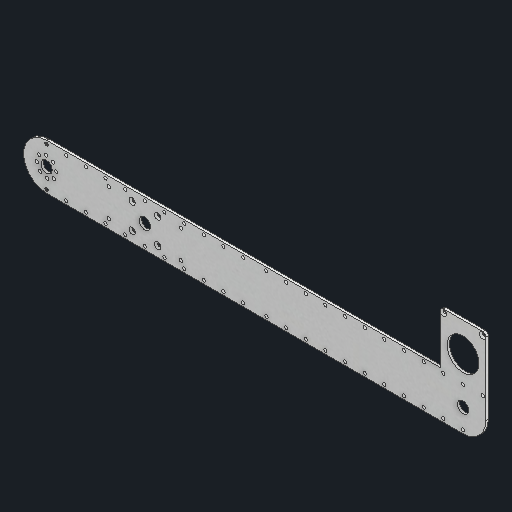
# Autodesk Inventor part: FirstStageArmBar1
Saved by Autodesk Inventor 2025 (Build 290162000, 162)
## iProperties
Created: 2023-11-22
Part Number: FirstStageArmBar1
Material: Aluminum 6061
Document SubType Name: Modeling
Designer: avsar
Density: 2.7 g/cm^3
Appearance: Paint
Mass: 273.267 g
Surface Area: 709.347 cm^2
Volume: 101.21 cm^3
Author: avsar
Autodesk Inventor part; units mm, degrees
ref_plane "YZ Plane" through (0, 0, 0) normal (1, 0, 0) x (0, 1, 0)
ref_plane "XZ Plane" through (0, 0, 0) normal (0, 1, 0) x (-1, 0, 0)
ref_plane "XY Plane" through (0, 0, 0) normal (0, 0, 1) x (1, 0, 0)
sketch "Sketch1" plane through (0, 0, 0) normal (0, 0, 1) x (1, 0, 0)
  line L0 (-254.2423, -28) -> (254.2423, -28)
  line L1 (282.2423, 0) -> (282.2423, 28)
  line L2 (282.2423, 28) -> (-254.2423, 28) construction
  line L3 (-282.2423, 0) -> (-282.2423, 0)
  line L4 (-282.2423, -28) -> (282.2423, 28) construction
  line L5 (282.2423, -28) -> (-282.2423, 28) construction
  arc A0 (-254.2423, 28) -> (-282.2423, 0) centre (-254.2423, 0) ccw
  arc A1 (-282.2423, 0) -> (-254.2423, -28) centre (-254.2423, 0) ccw
  circle A2 centre (-134.2423, 0) radius 7
  circle A3 centre (-149.7986, 15.5563) radius 2.1
  line L6 (-134.2423, 0) -> (-149.7986, 15.5563) construction
  line L7 (-134.2423, 0) -> (-254.2423, 0) construction
  circle A4 centre (-149.7986, -15.5563) radius 2.1
  circle A5 centre (-118.6859, -15.5563) radius 2.1
  circle A6 centre (-118.6859, 15.5563) radius 2.1
  arc A7 (254.2423, -28) -> (282.2423, 0) centre (254.2423, 0) ccw
  circle A8 centre (254.2423, 0) radius 7
  line L8 (282.2423, 28) -> (282.2423, 92)
  line L9 (282.2423, 92) -> (226.2423, 92)
  line L10 (226.2423, 92) -> (226.2423, 28)
  line L11 (226.2423, 28) -> (-254.2423, 28)
  circle A9 centre (254.2423, 56) radius 19.5
  circle A10 centre (-254.2423, 0) radius 7
  circle A11 centre (-263.1865, 8) radius 2
  circle A12 centre (-266.2237, -0.6677) radius 2
  circle A13 centre (-262.2423, -8.9443) radius 2
  circle A14 centre (-253.5746, -11.9814) radius 2
  circle A15 centre (-245.298, -8) radius 2
  circle A16 centre (-242.2609, 0.6677) radius 2
  circle A17 centre (-246.2423, 8.9443) radius 2
  circle A18 centre (-254.91, 11.9814) radius 2
  line L12 (-134.2423, 0) -> (254.2423, 56) construction
  point P0 (0, 0)
  point P1 (-282.2423, 0)
  dimension "d1" = 56
  dimension "d3" = 28
  dimension "d4" = 14
  dimension "d5" = 120
  dimension "d6" = 4.2
  dimension "d7" = 45
  dimension "d8" = 22
  dimension "d11" = 360
  dimension "d13" = 28
  dimension "d16" = 14
  dimension "d17" = 64
  dimension "d18" = 56
  dimension "d19" = 39
  dimension "d20" = 56
  dimension "d21" = 14
  dimension "d22" = 4
  dimension "d24" = 8
  dimension "d27" = 360
  dimension "d50" = 12
  dimension "d65" = 392.5
  constraints: 26 end point, 19 centre point, 9 point on line, 6 point on circle, 6 tangent, 3 perpendicular, 2 coincident, 2 midpoint, 2 parallel, 1 collinear, 1 concentric, 1 horizontal, 1 horizontal alignment, 1 vertical, 1 vertical alignment, 26 other
  measures "d1" distance of L4.end L5.start
  measures "d3" radius of A0
  measures "d4" diameter of A2
  measures "d5" distance of L6.start L7.end
  measures "d6" diameter of A3
  measures "d7" angle of L7 L6
  measures "d8" distance of L6.start L6.end
  measures "d13" radius of A7
  measures "d16" diameter of A8
  measures "d17" distance of L1.end L8.end
  measures "d18" distance of L8.end L9.end
  measures "d19" diameter of A9
  measures "d20" distance of L12.end A7.centre
  measures "d21" diameter of A10
  measures "d22" diameter of A11
  measures "d24" vertical distance of L7.end A11.centre
  measures "d50" distance of A11.centre L7.end
  measures "d65" distance of L6.start L12.end
extrude "Extrusion1" add sketch "Sketch1" along normal blind 3
sketch "Sketch2" plane through (0, 0, 3) normal (0, 0, 1) x (1, 0, 0)
  line L0 (226.2423, 28) -> (-254.2423, 28) construction
  circle A0 centre (-254.2423, 24) radius 2
  circle A1 centre (-230.2423, 24) radius 2
  circle A2 centre (-206.2423, 24) radius 2
  circle A3 centre (-182.2423, 24) radius 2
  circle A4 centre (-158.2423, 24) radius 2
  circle A5 centre (-134.2423, 24) radius 2
  circle A6 centre (-110.2423, 24) radius 2
  circle A7 centre (-86.2423, 24) radius 2
  circle A8 centre (-62.2423, 24) radius 2
  circle A9 centre (-38.2423, 24) radius 2
  circle A10 centre (-14.2423, 24) radius 2
  line L1 (0, 28) -> (0, -28) construction
  line L2 (-254.2423, -28) -> (254.2423, -28) construction
  circle A11 centre (254.2423, 24) radius 2
  circle A12 centre (230.2423, 24) radius 2
  circle A13 centre (206.2423, 24) radius 2
  circle A14 centre (182.2423, 24) radius 2
  circle A15 centre (158.2423, 24) radius 2
  circle A16 centre (134.2423, 24) radius 2
  circle A17 centre (110.2423, 24) radius 2
  circle A18 centre (86.2423, 24) radius 2
  circle A19 centre (62.2423, 24) radius 2
  circle A20 centre (38.2423, 24) radius 2
  circle A21 centre (14.2423, 24) radius 2
  arc A22 (-254.2423, 28) -> (-254.2423, -28) centre (-254.2423, 0) ccw construction
  arc A23 (254.2423, -28) -> (282.2423, 0) centre (254.2423, 0) ccw construction
  line L3 (-282.2423, 0) -> (282.2423, 0) construction
  line L4 (226.2423, -28) -> (-254.2423, -28) construction
  circle A24 centre (-254.2423, -24) radius 2
  circle A25 centre (-230.2423, -24) radius 2
  circle A26 centre (-206.2423, -24) radius 2
  circle A27 centre (-182.2423, -24) radius 2
  circle A28 centre (-158.2423, -24) radius 2
  circle A29 centre (-134.2423, -24) radius 2
  circle A30 centre (-110.2423, -24) radius 2
  circle A31 centre (-86.2423, -24) radius 2
  circle A32 centre (-62.2423, -24) radius 2
  circle A33 centre (-38.2423, -24) radius 2
  circle A34 centre (-14.2423, -24) radius 2
  circle A35 centre (62.2423, -24) radius 2
  circle A36 centre (38.2423, -24) radius 2
  circle A37 centre (14.2423, -24) radius 2
  circle A38 centre (86.2423, -24) radius 2
  circle A39 centre (110.2423, -24) radius 2
  circle A40 centre (134.2423, -24) radius 2
  circle A41 centre (158.2423, -24) radius 2
  circle A42 centre (182.2423, -24) radius 2
  circle A43 centre (206.2423, -24) radius 2
  circle A44 centre (230.2423, -24) radius 2
  circle A45 centre (254.2423, -24) radius 2
  circle A46 centre (230.2423, 88) radius 2.1
  line L5 (226.2423, 92) -> (226.2423, 28) construction
  line L6 (282.2423, 92) -> (226.2423, 92) construction
  circle A47 centre (278.2423, 88) radius 2.1
  line L7 (282.2423, 0) -> (282.2423, 92) construction
  circle A48 centre (278.2423, 24) radius 2.1
  point P0 (0, 0)
  point P1 (254.2423, 28)
  dimension "d29" = 4
  dimension "d30" = 4
  dimension "d33" = 24
  dimension "d38" = 4.2
  dimension "d39" = 4
  dimension "d40" = 4
  dimension "d41" = 4.2
  dimension "d42" = 4
  dimension "d43" = 4
  dimension "d56" = 4.2
  constraints: 47 centre point, 35 symmetric about line, 6 end point, 2 horizontal, 2 point on line, 2 vertical alignment, 1 horizontal alignment, 1 midpoint, 1 point on circle, 1 vertical, 53 other
  measures "d29" diameter of A0
  measures "d30" distance of L0.end A0.centre
  measures "d33" distance of A0.centre A1.centre
  measures "d38" diameter of A46
  measures "d39" distance from line of L5 A46.centre
  measures "d40" distance from line of L6 A46.centre
  measures "d41" diameter of A47
  measures "d42" distance from line of L6 A47.centre
  measures "d43" distance from line of L7 A47.centre
  measures "d56" diameter of A48
extrude "Extrusion2" cut sketch "Sketch2" against normal through all
sketch "Sketch3" plane through (0, 0, 3) normal (0, 0, 1) x (1, 0, 0)
  circle A0 centre (-134.2423, 0) radius 7 construction
  circle A1 centre (-90.2423, 17) radius 2.1
  line L0 (-134.2423, 0) -> (-127.2423, 0) construction
  circle A2 centre (-134.2423, 0) radius 7 construction
  line L1 (-134.2423, 0) -> (-134.2423, 7) construction
  circle A3 centre (-90.2423, -17) radius 2.1
  circle A4 centre (-178.2423, 17) radius 2.1
  circle A5 centre (-178.2423, -17) radius 2.1
  point P0 (0, 0)
  dimension "d51" = 4.2
  dimension "d52" = 44
  dimension "d53" = 17
  constraints: 4 centre point, 4 end point, 3 symmetric about line, 2 point on circle, 1 horizontal, 1 perpendicular, 3 other
  measures "d51" diameter of A1
  measures "d52" horizontal distance of A1.centre L0.start
  measures "d53" vertical distance of A1.centre L0.start
extrude "Extrusion3" cut sketch "Sketch3" against normal through all
fillet "Fillet1" radius 4 2 edges at (226.2423, 92, 1.5) (282.2423, 92, 1.5)
sketch "Sketch4" plane through (0, 0, 3) normal (0, 0, 1) x (1, 0, 0)
  circle A0 centre (-149.7986, 15.5563) radius 2.1 projected
  circle A1 centre (-118.6859, 15.5563) radius 2.1 projected
  circle A2 centre (-118.6859, -15.5563) radius 2.1 projected
  circle A3 centre (-149.7986, -15.5563) radius 2.1 projected
  point P0 (0, 0)
hole "Hole1" at (-149.7986, 15.5563, 3) at (-149.7986, -15.5563, 3) at (-118.6859, -15.5563, 3) at (-118.6859, 15.5563, 3) direction (0, 0, -1) diameter 4.2 end through all countersink diameter 8 countersink angle 90
sketch "Sketch5" plane through (0, 0, 0) normal (0, 0, -1) x (-1, 0, 0)
  circle A0 centre (178.2423, -17) radius 2.1 projected
  circle A1 centre (90.2423, -17) radius 2.1 projected
  circle A2 centre (90.2423, 17) radius 2.1 projected
  circle A3 centre (178.2423, 17) radius 2.1 projected
  circle A4 centre (158.2423, 24) radius 2 projected
  circle A5 centre (62.2423, 24) radius 2 projected
  circle A6 centre (62.2423, -24) radius 2 projected
  circle A7 centre (110.2423, -24) radius 2 projected
  circle A8 centre (206.2423, 24) radius 2 projected
  circle A9 centre (230.2423, -24) radius 2 projected
  circle A10 centre (-38.2423, -24) radius 2 projected
  circle A11 centre (-62.2423, -24) radius 2 projected
  circle A12 centre (-110.2423, 24) radius 2 projected
  circle A13 centre (-206.2423, 24) radius 2 projected
  circle A14 centre (-254.2423, -24) radius 2 projected
  circle A15 centre (-86.2423, -24) radius 2 projected
  circle A16 centre (-254.2423, 24) radius 2 projected
  circle A17 centre (-278.2423, 88) radius 2.1 projected
  circle A18 centre (-134.2423, 24) radius 2 projected
  circle A19 centre (-158.2423, -24) radius 2 projected
  circle A20 centre (-134.2423, -24) radius 2 projected
  circle A21 centre (-206.2423, -24) radius 2 projected
  circle A22 centre (182.2423, -24) radius 2 projected
  circle A23 centre (134.2423, -24) radius 2 projected
  circle A24 centre (38.2423, -24) radius 2 projected
  circle A25 centre (38.2423, 24) radius 2 projected
  circle A26 centre (134.2423, 24) radius 2 projected
  circle A27 centre (182.2423, 24) radius 2 projected
  circle A28 centre (86.2423, 24) radius 2 projected
  circle A29 centre (230.2423, 24) radius 2 projected
  circle A30 centre (86.2423, -24) radius 2 projected
  circle A31 centre (158.2423, -24) radius 2 projected
  circle A32 centre (206.2423, -24) radius 2 projected
  circle A33 centre (-182.2423, -24) radius 2 projected
  circle A34 centre (-62.2423, 24) radius 2 projected
  circle A35 centre (-86.2423, 24) radius 2 projected
  circle A36 centre (-182.2423, 24) radius 2 projected
  circle A37 centre (-38.2423, 24) radius 2 projected
  circle A38 centre (-14.2423, 24) radius 2 projected
  circle A39 centre (-14.2423, -24) radius 2 projected
  circle A40 centre (-230.2423, 24) radius 2 projected
  circle A41 centre (-158.2423, 24) radius 2 projected
  circle A42 centre (-230.2423, 88) radius 2.1 projected
  circle A43 centre (-110.2423, -24) radius 2 projected
  circle A44 centre (-230.2423, -24) radius 2 projected
  circle A45 centre (254.2423, -24) radius 2 projected
  circle A46 centre (254.2423, 24) radius 2 projected
  circle A47 centre (14.2423, -24) radius 2 projected
  circle A48 centre (14.2423, 24) radius 2 projected
  circle A49 centre (110.2423, 24) radius 2 projected
  circle A50 centre (-278.2423, 24) radius 2.1 projected
  arc A51 (-278.2423, 92) -> (-282.2423, 88) centre (-278.2423, 88) ccw projected
  line L0 (-282.2423, 0) -> (-282.2423, 88) projected
  arc A52 (-282.2423, 0) -> (-254.2423, -28) centre (-254.2423, 0) ccw projected
  line L1 (254.2423, -28) -> (-254.2423, -28) projected
  arc A53 (254.2423, -28) -> (254.2423, 28) centre (254.2423, 0) ccw projected
  line L2 (-226.2423, 28) -> (254.2423, 28) projected
  line L3 (-226.2423, 88) -> (-226.2423, 28) projected
  arc A54 (-226.2423, 88) -> (-230.2423, 92) centre (-230.2423, 88) ccw projected
  line L4 (-278.2423, 92) -> (-230.2423, 92) projected
  circle A55 centre (134.2423, 0) radius 7 projected
  circle A56 centre (149.7986, 15.5563) radius 2.1 projected
  circle A57 centre (149.7986, -15.5563) radius 2.1 projected
  circle A58 centre (118.6859, -15.5563) radius 2.1 projected
  circle A59 centre (118.6859, 15.5563) radius 2.1 projected
  circle A60 centre (-254.2423, 56) radius 19.5 projected
  circle A61 centre (242.2609, 0.6677) radius 2 projected
  circle A62 centre (254.91, 11.9814) radius 2 projected
  circle A63 centre (246.2423, 8.9443) radius 2 projected
  circle A64 centre (245.298, -8) radius 2 projected
  circle A65 centre (253.5746, -11.9814) radius 2 projected
  circle A66 centre (262.2423, -8.9443) radius 2 projected
  circle A67 centre (266.2237, -0.6677) radius 2 projected
  circle A68 centre (263.1865, 8) radius 2 projected
  circle A69 centre (254.2423, 0) radius 7 projected
  circle A70 centre (-254.2423, 0) radius 7 projected
  point P0 (0, 0)
hole "Hole2" at (-254.2423, 24, 0) at (-254.2423, -24, 0) direction (0, 0, 1) diameter 4.12 end through all countersink diameter 8 countersink angle 90
hole "Hole3" at (230.2423, 88, 3) at (278.2423, 88, 3) direction (0, 0, -1) diameter 4.12 end through all countersink diameter 8 countersink angle 90
equation "\"d3\" = 0.5 * d1"
equation "\"d13\" = d3"
body "Solid1"
